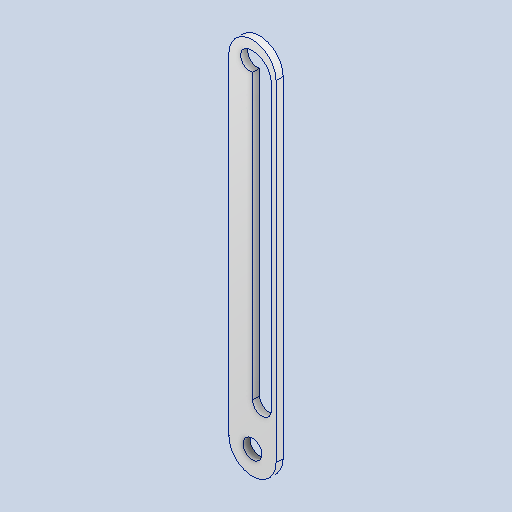
# Autodesk Inventor part: držák
Saved by Autodesk Inventor 2023 (Build 270158000, 158)
## iProperties
Created: 2023-04-03
Part Number: držák
Material: Aluminum 6061
Document SubType Name: Modeling
Designer: lukyv
Density: 2.7 g/cm^3
Appearance: Aluminum - Flat
Mass: 2.02022 g
Surface Area: 14.834 cm^2
Volume: 0.748229 cm^3
Author: lukyv
Autodesk Inventor part; units mm, degrees
ref_plane "YZ Plane" through (0, 0, 0) normal (1, 0, 0) x (0, 1, 0)
ref_plane "XZ Plane" through (0, 0, 0) normal (0, 1, 0) x (-1, 0, 0)
ref_plane "XY Plane" through (0, 0, 0) normal (0, 0, 1) x (1, 0, 0)
sketch "Sketch1" plane through (0, 0, 0) normal (0, 0, 1) x (1, 0, 0)
  line L0 (-9.2249, 16.9065) -> (-9.2249, 86.9065)
  line L1 (0.7751, 86.9065) -> (0.7751, 16.9065)
  arc A0 (-9.2249, 16.9065) -> (-4.2249, 11.9065) centre (-4.2249, 16.9065) ccw
  arc A1 (-4.2249, 11.9065) -> (0.7751, 16.9065) centre (-4.2249, 16.9065) ccw
  arc A2 (0.7751, 86.9065) -> (-4.2249, 91.9065) centre (-4.2249, 86.9065) ccw
  arc A3 (-4.2249, 91.9065) -> (-9.2249, 86.9065) centre (-4.2249, 86.9065) ccw
  circle A4 centre (-4.2249, 16.9065) radius 2
  line L2 (-4.2249, 11.9065) -> (-4.2249, 91.9065) construction
  line L3 (0.7751, 16.9065) -> (-9.2249, 16.9065) construction
  point P0 (0, 0)
  point P1 (-9.2249, 91.9065)
  point P2 (-9.2249, 11.9065)
  point P3 (0.7751, 91.9065)
  point P4 (-4.2249, 11.9065)
  dimension "d0" = 10
  dimension "d1" = 80
  dimension "d2" = 5
  dimension "d3" = 4
  constraints: 8 end point, 8 point on circle, 5 centre point, 5 point on line, 4 tangent, 3 equal radius, 1 midpoint, 1 parallel, 1 vertical, 13 other
  measures "d0" distance of point (-9.225, 91.907) point (0.775, 91.907)
  measures "d1" distance of point (-9.225, 11.907) point (-9.225, 91.907)
  measures "d2" radius of A0
  measures "d3" diameter of A4
extrude "Extrusion1" add sketch "Sketch1" along normal blind 1.5
sketch "Sketch2" plane through (0, 0, 1.5) normal (0, 0, 1) x (1, 0, 0)
  circle A0 centre (-4.7249, 87.843) radius 2
  line L0 (-9.2249, 86.9065) -> (-9.2249, 16.9065) projected
  line L1 (0.7751, 16.9065) -> (0.7751, 86.9065) projected
  line L2 (0.7751, 85.9065) -> (-9.2249, 85.9065) construction
  circle A1 centre (-4.2249, 85.9065) radius 4
  line L3 (-4.2249, 85.9065) -> (-4.2249, 25.9065)
  line L4 (-4.2249, 25.9065) -> (-0.2249, 25.9065)
  line L5 (-0.2249, 25.9065) -> (-0.2249, 85.9065)
  circle A2 centre (-2.2249, 25.9065) radius 2
  arc A3 (0.7751, 86.9065) -> (-9.2249, 86.9065) centre (-4.2249, 86.9065) ccw projected
  point P0 (0, 0)
  point P1 (-5.2249, 89.7795)
  point P2 (-4.2249, 81.9065)
  point P3 (-4.2249, 91.9065)
  dimension "d6" = 4
  dimension "d8" = 8
  dimension "d7" = 4.5
  dimension "d9" = 4
  dimension "d10" = 60
  dimension "d13" = 6
  constraints: 8 end point, 3 point on line, 2 midpoint, 2 perpendicular, 1 point on circle, 9 other
  measures "d7" distance from line of L0 point (-4.725, 87.843)
  measures "d9" distance of L3.end L4.end
  measures "d10" distance of L3.start L3.end
  measures "d13" distance of point (-4.225, 91.907) L3.start
extrude "Extrusion2" cut sketch "Sketch2" against normal blind 1.5 contours A0 | A0 A1 L3 | A1 L5 A2 L3 | A2 L4 | L4 A2 picked at (-3.9282, 83.2733)
body "Solid1"
